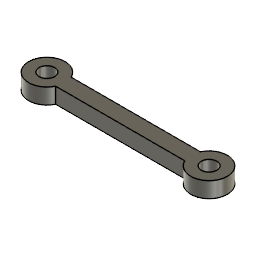
Simple gripper_Link (Autodesk Fusion 360 design; units mm, degrees)
Autodesk Fusion 360 part; units mm, degrees
note: some values were not read from the file. Set by a fixed rule: which sketch regions a step uses.
sketch "Sketch1" plane through (0, 0, 0) normal (0, 0, 1) x (1, 0, 0)
  circle A0 centre (-30.1129, -14.4636) radius 3.5
  circle A1 centre (-30.1129, -14.4636) radius 1.5
  line L0 (-30.1129, -14.4636) -> (0.8871, -14.4636)
  line L1 (-14.6129, -4.9636) -> (-14.6129, -23.9636) construction
  circle A2 centre (0.8871, -14.4636) radius 3.5
  circle A3 centre (0.8871, -14.4636) radius 1.5
  line L2 (-26.9506, -12.9636) -> (-2.2752, -12.9636)
  line L3 (-26.9506, -15.9636) -> (-2.2752, -15.9636)
  point P0 (0.8871, -14.4636)
  dimension "d1" = 7
  dimension "d2" = 3
  dimension "d3" = 31
  dimension "d4" = 1.5
  constraint concentric A0 A1
  constraint coincident A0.centre A1.centre
  constraint horizontal L0
  constraint vertical L1
  constraint midpoint L0 L1
  constraint symmetric A0 L1 A2
  constraint symmetric A1 L1 A3
  constraint symmetric A0.centre L1 P0
  constraint coincident A0 L2.start
  constraint coincident A2 L2.end
  constraint perpendicular L1 L2
  constraint symmetric L0 L2.start L3.start
  constraint symmetric L0 L2.end L3.end
  measures "d1" diameter of A0
  measures "d2" diameter of A1
  measures "d3" distance of A0.centre P0
  measures "d4" distance of L0 L2
extrude "Extrude1" add sketch "Sketch1" along normal blind 3
